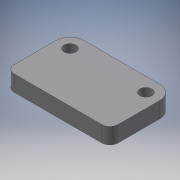
# Autodesk Inventor part: XY-Endstop holder
Saved by Autodesk Inventor 2016 (Build 200138000, 138)
## iProperties
Created: 2015-08-05
Part Number: XY-Endstop holder
Material: Generic
Document SubType Name: Modeling
Designer: Mathias L. Kjeldgaard
Density: 1 g/cm^3
Appearance: Default
Author: Mathias L. Kjeldgaard
Autodesk Inventor part; units mm, degrees
ref_plane "YZ Plane" through (0, 0, 0) normal (1, 0, 0) x (0, 1, 0)
ref_plane "XZ Plane" through (0, 0, 0) normal (0, 1, 0) x (-1, 0, 0)
ref_plane "XY Plane" through (0, 0, 0) normal (0, 0, 1) x (1, 0, 0)
sketch "Sketch1" plane through (0, 0, 0) normal (0, 0, 1) x (1, 0, 0)
  circle A0 centre (-9.5, 0) radius 1.5
  circle A1 centre (9.5, 0) radius 1.5
  line L0 (8, 3.8632) -> (8, -14.6027) construction
  line L1 (11, -2.0672) -> (11, -20.5331) construction
  line L2 (-8, 0.17) -> (-8, -13.1822) construction
  line L3 (-11, -0.1851) -> (-11, -13.1822) construction
  line L4 (19.0881, 0) -> (-23.3125, 0) construction
  arc A2 (-9.5, 3.5) -> (-13, 0) centre (-9.5, 0) ccw
  arc A3 (13, 0) -> (9.5, 3.5) centre (9.5, 0) ccw
  line L5 (9.5, 3.5) -> (-9.5, 3.5)
  line L6 (-14.1747, 14.7489) -> (-2.6119, 14.7489) construction
  line L7 (-2.6119, 14.7489) -> (-2.6119, 6.4897) construction
  line L8 (-2.6119, 6.4897) -> (-14.1747, 6.4897) construction
  line L9 (-14.1747, 6.4897) -> (-14.1747, 14.7489) construction
  line L10 (-13, 0) -> (-13, -10.5)
  line L11 (-11, -12.5) -> (11, -12.5)
  line L12 (13, -10.5) -> (13, 0)
  arc A4 (-13, -10.5) -> (-11, -12.5) centre (-11, -10.5) ccw
  arc A5 (11, -12.5) -> (13, -10.5) centre (11, -10.5) ccw
  point P0 (0, 0)
  dimension "d0" = 3
  dimension "d1" = 3
  dimension "d2" = 16
  dimension "d3" = 22
  dimension "d6" = 9.5
  dimension "d7" = 2
  dimension "d8" = 2
  dimension "d9" = 16
  dimension "d10" = 2
  constraints: 18 end point, 11 tangent, 8 point on circle, 6 centre point, 5 parallel, 5 point on line, 3 perpendicular, 2 coincident, 1 equal radius, 1 vertical, 2 other
  measures "d0" diameter of A1
  measures "d1" diameter of A0
  measures "d2" distance between parallel lines of L0 L2
  measures "d3" distance between parallel lines of L1 L3
  measures "d6" distance of point (0, 0) A1.centre
  measures "d7" radial gap between concentric circles of A1 A3
  measures "d8" radial gap between concentric circles of A0 A2
  measures "d9" distance between parallel lines of L5 L11
  measures "d10" radius of A4
extrude "Extrusion1" add sketch "Sketch1" along normal blind 2
equation "\"d0\" = d1"
body "Solid1"
